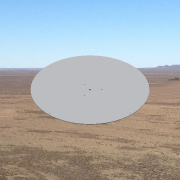
# Autodesk Inventor part: 2f1bd
Saved by Autodesk Inventor 2014 SP1 (Build 180222100, 222)
## iProperties
Company: HERA Project
Created: 2013-05-22
Part Number: 2f1bd
Material: Aluminum 6061
Document SubType Name: Modeling
Designer: Rich Bradley
Density: 2.71 g/cm^3
Description: Feed bottom disk
Mass: 2472.03 g
Surface Area: 5814.47 cm^2
Volume: 912.187 cm^3
Appearance: Aluminum - Flat
Translation Standard: STEP AP214IS
FileName: C:/Users/Dave/Desktop/PAPER/paperElement.step
PostProcessor: Build: 138, Release: 2013 RTM - Date: Thu 03/01/2012
Sent Units: millimeter
Uncertainty: 2.54e-05
Author: David DeBoer
Title: Feed bottom disk
Autodesk Inventor part; units mm, degrees
ref_plane "YZ Plane" through (0, 0, 0) normal (1, 0, 0) x (0, 1, 0)
ref_plane "XZ Plane" through (0, 0, 0) normal (0, 1, 0) x (-1, 0, 0)
ref_plane "XY Plane" through (0, 0, 0) normal (0, 0, 1) x (1, 0, 0)
sketch "Sketch1" plane through (0, 0, 0) normal (0, 1, 0) x (-1, 0, 0)
  circle A0 centre (0, 0) radius 304.8
  dimension "d0" = 609.6
  constraints: 1 centre point, 1 coincident
  measures "d0" diameter of A0
extrude "Extrusion1" add sketch "Sketch1" along normal blind 3.175
sketch "Sketch2" plane through (0, 3.175, 0) normal (0, 1, 0) x (1, 0, 0)
  circle A0 centre (0, 0) radius 304.8 projected
  circle A1 centre (0, 0) radius 6.35
  dimension "d3" = 12.7
  constraints: 1 centre point, 1 coincident
  measures "d3" diameter of A1
extrude "Extrusion2" cut sketch "Sketch2" against normal blind 3.175 contours A1
sketch "Sketch3" plane through (0, 3.175, 0) normal (0, 1, 0) x (1, 0, 0)
  circle A0 centre (0, 0) radius 6.35 projected
  circle A1 centre (0, 292.1) radius 4.6302
  dimension "d6" = 292.1
  constraints: 1 centre point
  measures "d6" distance of A1.centre A0.centre
hole "Hole1" at (0, 3.175, -292.1) direction (0, -1, 0) diameter 4.4958 end through all countersink diameter 8.4328 countersink angle 82
pattern_circular "Circular Pattern1" count 4 over 360 about axis through (0, 3.175, 0) along (0, -1, 0) of "Hole1"
sketch "Sketch9" plane through (0, 3.175, 0) normal (0, 1, 0) x (1, 0, 0)
  circle A0 centre (0, 0) radius 304.8 projected
  line L0 (0, 0) -> (14.7527, -55.0578) construction
  line L1 (0, 0) -> (57, 0) construction
  line L2 (0, 0) -> (-55.0578, 14.7527) construction
  line L3 (0, 0) -> (57, 0) construction
  circle A1 centre (42.4264, 42.4264) radius 7.377
  circle A2 centre (14.7527, -55.0578) radius 7.6366
  circle A3 centre (-55.0578, 14.7527) radius 7.2502
  circle A4 centre (0, 0) radius 6.35 projected
  line L4 (0, 0) -> (42.4264, 42.4264) construction
  line L5 (0, 0) -> (60, 0) construction
  dimension "d85" = 57
  dimension "d86" = 75
  dimension "d87" = 57
  dimension "d88" = 195
  dimension "d96" = 60
  dimension "d97" = 45
  constraints: 12 end point, 4 coincident, 3 centre point, 3 equal length, 3 horizontal
  measures "d85" distance of L0.start L0.end
  measures "d86" angle of L0 L1
  measures "d87" distance of L0.start L2.end
  measures "d96" distance of L4.start L4.end
  measures "d97" angle of L5 L4
hole "Hole7" at (-55.0578, 3.175, -14.7527) at (42.4264, 3.175, -42.4264) at (14.7527, 3.175, 55.0578) direction (0, -1, 0) diameter 6.6 end through all clearance for "Flat Head Machine Screw" size "M6" standard "Ansi Metric M Profile"
body "Solid2"
